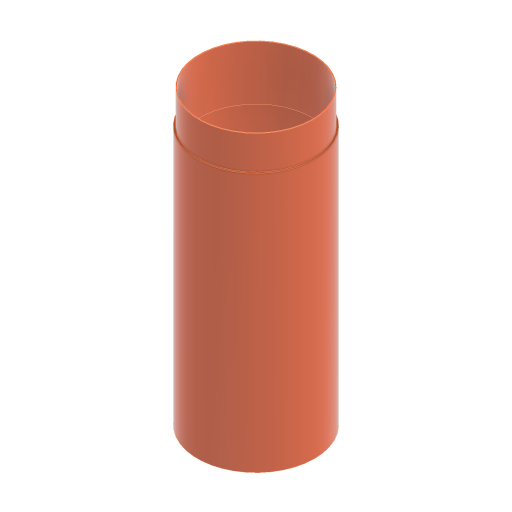
# Autodesk Inventor part: Engine skin
Saved by Autodesk Inventor 2024 (Build 280153000, 153)
## iProperties
Created: 2023-12-30
Part Number: Engine skin
Material: Plastic, Opaque White
Document SubType Name: Modeling
Designer: Jamie
Density: 0.952 g/cm^3
Appearance: Smooth - Light Orange
Author: Jamie
Autodesk Inventor part; units mm, degrees
ref_plane "XZ Plane" through (0, 0, 0) normal (0, 1, 0) x (-1, 0, 0)
ref_plane "XY Plane" through (0, 0, 0) normal (0, 0, 1) x (1, 0, 0)
sketch "Sketch1" plane through (0, 0, 0) normal (0, 1, 0) x (-1, 0, 0)
  circle A0 centre (0, 0) radius 35
  circle A1 centre (0, 0) radius 34.5
  dimension "d0" = 70
  dimension "d1" = 69
  constraints: 2 centre point, 2 coincident
  measures "d0" diameter of A0
  measures "d1" diameter of A1
extrude "Extrusion1" add sketch "Sketch1" along normal blind 155
ref_plane "Work Plane2" through (35, 0, 0) normal (1, 0, 0) x (0, 1, 0)
sketch "Sketch5" plane through (0, 155, 0) normal (0, 1, 0) x (1, 0, 0)
  circle A0 centre (0, 0) radius 34
  circle A1 centre (0, 0) radius 33.5
  dimension "d44" = 68
  dimension "d45" = 67
  constraints: 2 centre point, 2 coincident
  measures "d44" diameter of A0
  measures "d45" diameter of A1
extrude "Extrusion3" add sketch "Sketch5" along normal blind 20
sketch "Sketch6" plane through (0, 155, 0) normal (0, -1, 0) x (1, 0, 0)
  circle A0 centre (0, 0) radius 33.5
  circle A1 centre (0, 0) radius 34.5 projected
  circle A2 centre (0, 0) radius 35
  constraints: 2 centre point, 2 coincident
extrude "Extrusion4" add sketch "Sketch6" along normal blind 12.5 contours A1
ref_plane "Work Plane4" through (34, 0, 0) normal (1, 0, 0) x (0, 1, 0)
ref_plane "Work Plane5" through (0, 8, 0) normal (0, -1, 0) x (1, 0, 0)
sketch "Sketch11" plane through (0, 8, 0) normal (0, -1, 0) x (1, 0, 0)
  line L0 (0, 0) -> (37.8059, -6.6662) construction
  line L1 (37.8059, 6.6662) -> (0, 0) construction
  line L2 (0, 0) -> (37.8692, 0) construction
  arc A0 (33.9759, -5.9909) -> (33.9759, 5.9909) centre (0, 0) ccw
  arc A1 (31.0214, -5.4699) -> (31.0214, 5.4699) centre (0, 0) ccw
  line L3 (31.0214, 5.4699) -> (33.9759, 5.9909)
  line L4 (31.0214, -5.4699) -> (33.9759, -5.9909)
  dimension "d94" = 10
  dimension "d95" = 10
  dimension "d96" = 34.5
  dimension "d97" = 31.5
  constraints: 10 end point, 4 point on circle, 3 point on line, 2 centre point, 2 coincident, 2 collinear
  measures "d94" angle of L1 L2
  measures "d95" angle of L0 L2
  measures "d96" radius of A0
  measures "d97" radius of A1
extrude "Extrusion5" add sketch "Sketch11" against normal blind 4
chamfer "Chamfer1" distance 1.5 angle 60 2 edges at (32.4987, 8, -5.7304) (32.4987, 8, 5.7304) measured on face at (32.5855, 8, -5.238) measured on face at (32.5855, 8, 5.238)
pattern_circular "Circular Pattern4" count 3 over 360 about axis through (0, 0, 0) along (0, 1, 0) of "Extrusion5", "Chamfer1"
ref_plane "Work Plane6" through (0, 25, 0) normal (0, -1, 0) x (1, 0, 0)
sketch "Sketch12" plane through (0, 25, 0) normal (0, -1, 0) x (1, 0, 0)
  circle A0 centre (0, 0) radius 34.5
  constraints: 1 centre point, 1 coincident
extrude "Extrusion6" add sketch "Sketch12" along normal blind 4
body "Solid1"
